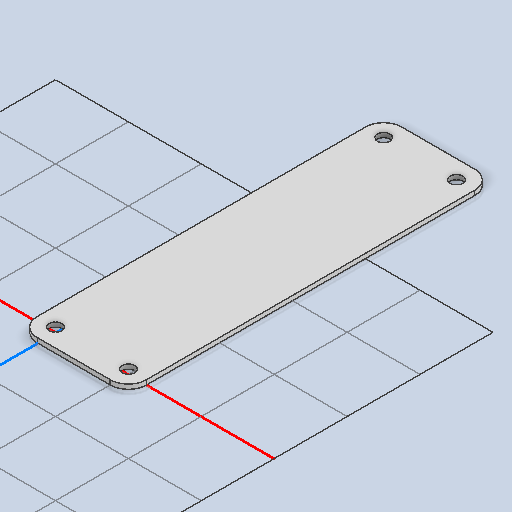
# Autodesk Inventor part: Brace Gusset
Saved by Autodesk Inventor 2026 (Build 300175000, 175)
## iProperties
Created: 2025-04-12
Part Number: Brace Gusset
Material: Generic
Document SubType Name: Modeling
Designer: avere
Density: 1 g/cm^3
Appearance: Default
Author: avere
Autodesk Inventor part; units mm, degrees
ref_plane "YZ Plane" through (0, 0, 0) normal (1, 0, 0) x (0, 1, 0)
ref_plane "XZ Plane" through (0, 0, 0) normal (0, 1, 0) x (-1, 0, 0)
ref_plane "XY Plane" through (0, 0, 0) normal (0, 0, 1) x (1, 0, 0)
sketch "main" plane through (0, 0, 0) normal (0, 0, 1) x (1, 0, 0)
  circle A0 centre (-11.9584, 56.4908) radius 2.1844
  circle A1 centre (13.4416, 56.4908) radius 2.1844
  circle A2 centre (13.4416, -57.8092) radius 2.1844
  circle A3 centre (-11.9584, -57.8092) radius 2.1844
  arc A4 (19.7916, 56.4908) -> (13.4416, 62.8408) centre (13.4416, 56.4908) ccw
  arc A5 (-11.9584, 62.8408) -> (-18.3084, 56.4908) centre (-11.9584, 56.4908) ccw
  arc A6 (-18.3084, -57.8092) -> (-11.9584, -64.1592) centre (-11.9584, -57.8092) ccw
  arc A7 (13.4416, -64.1592) -> (19.7916, -57.8092) centre (13.4416, -57.8092) ccw
  line L0 (13.4416, 62.8408) -> (-11.9584, 62.8408)
  line L1 (-18.3084, 56.4908) -> (-18.3084, -57.8092)
  line L2 (-11.9584, -64.1592) -> (13.4416, -64.1592)
  line L3 (19.7916, -57.8092) -> (19.7916, 56.4908)
  point P0 (0.7416, -0.6592)
  dimension "d0" = 12.7
  dimension "d1" = 12.7
  dimension "d2" = 12.7
  dimension "d3" = 12.7
  measures "d0" diameter of A4
  measures "d1" diameter of A5
  measures "d2" diameter of A6
  measures "d3" diameter of A7
sketch "Sketch1" plane through (0, 0, 0) normal (0, 1, 0) x (-1, 0, 0)
  circle A0 centre (-25.4, 0) radius 2.1844
  circle A1 centre (0, 0) radius 2.1844
  circle A2 centre (0, -114.3) radius 2.1844
  circle A3 centre (-25.4, -114.3) radius 2.1844
  arc A4 (6.35, 0) -> (0, 6.35) centre (0, 0) ccw
  arc A5 (-25.4, 6.35) -> (-31.75, 0) centre (-25.4, 0) ccw
  arc A6 (-31.75, -114.3) -> (-25.4, -120.65) centre (-25.4, -114.3) ccw
  arc A7 (0, -120.65) -> (6.35, -114.3) centre (0, -114.3) ccw
  line L0 (0, 6.35) -> (-25.4, 6.35)
  line L1 (-31.75, 0) -> (-31.75, -114.3)
  line L2 (-25.4, -120.65) -> (0, -120.65)
  line L3 (6.35, -114.3) -> (6.35, 0)
  constraints: 1 other
extrude "Extrusion1" add sketch "Sketch1" along normal blind 1.5875
body "Solid1"
